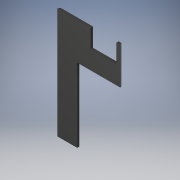
# Autodesk Inventor part: BA03
Saved by Autodesk Inventor 2017 (Build 210142000, 142)
## iProperties
Created: 2018-10-18
Part Number: BA03
Material: ABS Plastic
Document SubType Name: Modeling
Designer: Dell
Density: 1.06 g/cm^3
Appearance: Smooth - Black
Author: Dell
Autodesk Inventor part; units mm, degrees
ref_plane "YZ Plane" through (0, 0, 0) normal (1, 0, 0) x (0, 1, 0)
ref_plane "XZ Plane" through (0, 0, 0) normal (0, 1, 0) x (-1, 0, 0)
ref_plane "XY Plane" through (0, 0, 0) normal (0, 0, 1) x (1, 0, 0)
sketch "Sketch1" plane through (0, 0, 0) normal (0, 0, 1) x (1, 0, 0)
  line L0 (0, 0) -> (292.1, 0)
  line L1 (292.1, 0) -> (292.1, -177.8)
  line L2 (292.1, -177.8) -> (0, -177.8)
  line L3 (0, -177.8) -> (0, 0)
  dimension "d0" = 292.1
  dimension "d1" = 177.8
  constraints: 8 end point, 2 parallel, 1 horizontal, 1 perpendicular
  measures "d0" distance of L1.end L2.end
  measures "d1" distance of L0.end L1.end
extrude "Extrusion1" add sketch "Sketch1" along normal blind 10
sketch "Sketch2" plane through (0, 0, 0) normal (0, 1, 0) x (1, 0, 0)
  line L0 (292.1, -10) -> (0, -10) projected
  line L1 (0, -10) -> (-5.7735, -10)
  line L2 (-5.7735, -10) -> (0, 0)
  line L3 (0, 0) -> (0, -10) projected
  line L4 (0, 0) -> (0, -10) projected
  line L5 (0, -10) -> (0, 0)
  line L6 (292.1, -10) -> (297.8735, -10)
  line L7 (292.1, 0) -> (292.1, -10) projected
  line L8 (297.8735, -10) -> (292.1, 0)
  line L9 (292.1, 0) -> (292.1, -10)
  dimension "d4" = 30
  dimension "d5" = 60
  constraints: 12 end point, 2 collinear, 2 horizontal
  measures "d4" angle of L3 L2
  measures "d5" angle of L6 L8
extrude "Extrusion2" add sketch "Sketch2" against normal blind 177.8
sketch "Sketch3" plane through (0, 0, 10) normal (0, 0, 1) x (1, 0, 0)
  line L0 (79.2265, -88.9) -> (279.2265, -88.9)
  line L1 (279.2265, -88.9) -> (279.2265, 0)
  line L2 (279.2265, 0) -> (79.2265, 0)
  line L3 (79.2265, 0) -> (79.2265, -88.9)
  line L4 (-5.7735, 0) -> (297.8735, 0) projected
  line L5 (79.2265, -88.9) -> (190.7027, -88.9)
  line L6 (121.05, 0) -> (79.2265, 0)
  line L7 (79.2265, 0) -> (79.2265, -88.9)
  line L8 (279.2265, 0) -> (169.304, 0)
  line L9 (154.2265, -88.9) -> (279.2265, -88.9)
  line L10 (279.2265, -88.9) -> (279.2265, 0)
  line L11 (79.2265, 0) -> (154.2265, 0)
  line L12 (154.2265, 0) -> (154.2265, -88.9)
  line L13 (154.2265, -88.9) -> (79.2265, -88.9)
  line L14 (79.2265, -88.9) -> (79.2265, 0)
  line L15 (279.2265, 0) -> (279.2265, -88.9)
  line L16 (279.2265, -88.9) -> (279.2265, 0)
  line L17 (-5.7735, 0) -> (-5.7735, -177.8) projected
  point P0 (0, 0)
  point P1 (279.2265, -44.45)
  point P2 (146.05, 0)
  point P3 (146.05, 0)
  dimension "d8" = 200
  dimension "d9" = 88.9
  dimension "d14" = 75
  dimension "d33" = 85
  constraints: 32 end point, 6 parallel, 5 midpoint, 4 horizontal, 4 point on line, 2 coincident, 2 perpendicular, 2 vertical, 1 collinear, 4 other
  measures "d8" distance of L1.end L2.end
  measures "d9" distance of L0.end L1.end
  measures "d14" distance between parallel lines of L3 L12
  measures "d33" distance between parallel lines of L17 L14
extrude "Extrusion3" cut sketch "Sketch3" against normal through all contours L12 L2 L1 L0
sketch "Sketch5" plane through (0, 0, 10) normal (0, 0, 1) x (1, 0, 0)
  line L0 (297.8735, -177.8) -> (-5.7735, -177.8) projected
  line L1 (-5.7735, -177.8) -> (89.4765, -177.8)
  line L2 (89.4765, -177.8) -> (89.4765, -533.4)
  line L3 (89.4765, -533.4) -> (-5.7735, -533.4)
  line L4 (-5.7735, -533.4) -> (-5.7735, -177.8)
  point P0 (0, 0)
  dimension "d23" = 95.25
  dimension "d24" = 355.6
  constraints: 8 end point, 2 parallel, 1 horizontal, 1 perpendicular
  measures "d23" distance between parallel lines of L2 L4
  measures "d24" distance of L3.end L0.end
extrude "Extrusion5" add sketch "Sketch5" against normal blind 10
sketch "Sketch6" plane through (-5.7735, -177.8, 0) normal (0, 1, 0) x (1, 0, 0)
  line L0 (0, -10) -> (5.7735, 0) projected
  line L1 (0, 0) -> (5.7735, 0) projected
  line L2 (0, -10) -> (0, 0) projected
  point P0 (5.7735, 0)
extrude "Extrusion6" cut sketch "Sketch6" against normal through all
body "Solid1"
